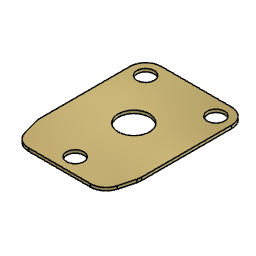
smb electrode top ground v14 (Autodesk Fusion 360 design; units mm, degrees)
Autodesk Fusion 360 part; units mm, degrees
sketch "Sketch1" plane through (0, 0, 0) normal (0, 1, 0) x (1, 0, 0)
  circle A0 centre (-4.5, 13.5) radius 1.1
  circle A1 centre (4.5, 13.5) radius 1.1
  line L0 (0, -20) -> (0, -2.5) construction
  circle A2 centre (0, 0) radius 1.1
  circle A3 centre (0, 7.5) radius 2
  line L1 (-6.5, -2) -> (6.5, -2)
  line L2 (6.5, -2) -> (6.5, 15.5)
  line L3 (-6.5, -2) -> (-6.5, 15.5)
  line L4 (6.5, 15.5) -> (-6.5, 15.5)
  line L5 (-5.5, -2) -> (-6.5, 1.7321)
  line L6 (5.5, -2) -> (6.5, 1.7321)
  dimension "d1" = 2.2
  dimension "d2" = 2.2
  dimension "d3" = 9
  dimension "d4" = 13.5
  dimension "d5" = 2.2
  dimension "d6" = 7.5
  dimension "d7" = 4
  dimension "d8" = 13
  dimension "d9" = 2
  dimension "d10" = 2
  dimension "d15" = 30
  dimension "d16" = 11
  constraint horizontal A0.centre A1.centre
  constraint symmetric A0.centre A1.centre L0
  constraint coincident A2.centre origin
  constraint vertical A2.centre A3.centre
  constraint horizontal L1
  constraint perpendicular L1 L2
  constraint perpendicular L1 L3
  constraint perpendicular L2 L4
  constraint coincident L1 L5.start
  constraint coincident L3 L5.end
  constraint coincident L1 L6.start
  constraint coincident L2 L6.end
  constraint symmetric L0 L5 L6
  measures "d1" diameter of A0
  measures "d2" diameter of A1
  measures "d3" horizontal distance of A0.centre A1.centre
  measures "d4" vertical distance of A2.centre A1.centre
  measures "d5" diameter of A2
  measures "d6" distance of A2.centre A3.centre
  measures "d7" diameter of A3
  measures "d8" distance of L1.start L1.end
  measures "d9" distance of A2.centre L1
  measures "d10" distance of A1.centre L4
  measures "d15" angle of L5 L6
  measures "d16" distance of L5.start L6.start
extrude "Extrude1" add sketch "Sketch1" along normal blind 0.38 contours L1 L2 L3 L4 L5 L6
fillet "Fillet1" radius 2 6 edges at (-6.5, 0.19, -15.5) (6.5, 0.19, -15.5) (-5.5, 0.19, 2) (-6.5, 0.19, -1.7321) (5.5, 0.19, 2) (6.5, 0.19, -1.7321)
